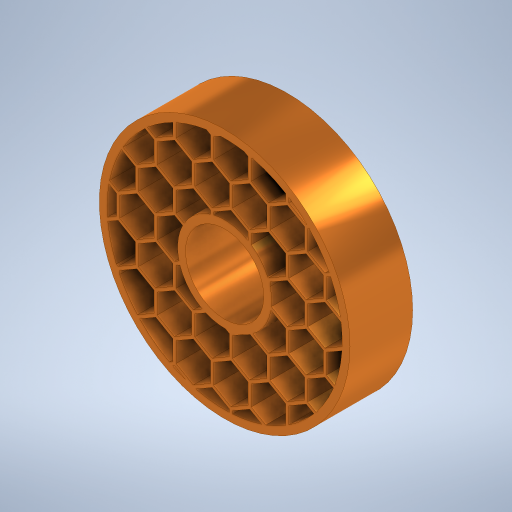
# Autodesk Inventor part: Idea3
Saved by Autodesk Inventor 2024.2 (Build 282272000, 272)
## iProperties
Created: 2025-07-14
Part Number: Idea3
Material: Generic
Document SubType Name: Modeling
Designer: Admin
Density: 1 g/cm^3
Appearance: Metal 1600F Hot
Author: Admin
Autodesk Inventor part; units mm, degrees
ref_plane "YZ Plane" through (0, 0, 0) normal (1, 0, 0) x (0, 1, 0)
ref_plane "XZ Plane" through (0, 0, 0) normal (0, 1, 0) x (-1, 0, 0)
ref_plane "XY Plane" through (0, 0, 0) normal (0, 0, 1) x (1, 0, 0)
sketch "Sketch1" plane through (0, 0, 0) normal (0, 0, 1) x (1, 0, 0)
  circle A0 centre (0, 0) radius 12.5
  circle A1 centre (0, 0) radius 40
  circle A2 centre (0, 0) radius 37.5
  circle A3 centre (0, 0) radius 15
  line L0 (0, 15) -> (0, 37.5) construction
  dimension "d2" = 75
  dimension "d3" = 30
  dimension "d0" = 25
  dimension "d1" = 80
  dimension "d4" = 22.5
  constraints: 4 coincident, 2 centre point, 2 end point, 2 vertical alignment, 1 vertical, 4 other
  measures "d0" diameter of A0
  measures "d1" diameter of A1
  measures "d4" distance of L0.start L0.end
extrude "Extrusion1" add sketch "Sketch1" along normal blind 20
sketch "Sketch2" plane through (0, 0, 20) normal (0, 0, 1) x (1, 0, 0)
  line L0 (40, -40) -> (-40, -40)
  line L1 (-40, -40) -> (-40, 40)
  line L2 (-40, 40) -> (40, 40)
  line L3 (40, 40) -> (40, -40)
  circle A0 centre (0, 0) radius 12.5 projected
  line L4 (40, -40) -> (-40, 40) construction
  line L5 (-40, -40) -> (40, 40) construction
  line L6 (-40, 40) -> (-64, 40) construction
  line L7 (-64, 40) -> (-64, -40) construction
  line L8 (-64, -40) -> (-40, -40)
  line L9 (-40, -40) -> (-40, 40)
  line L10 (-58, 40) -> (-52, 36.5359)
  line L11 (-52, 36.5359) -> (-52, 29.6077)
  line L12 (-58, 26.1436) -> (-64, 29.6077)
  line L13 (-64, 29.6077) -> (-64, 36.5359)
  line L14 (-64, 36.5359) -> (-58, 40)
  line L15 (-58, 33.0718) -> (-52, 22.6795) construction
  line L16 (-52, 29.6077) -> (-46, 26.1436)
  line L17 (-46, 26.1436) -> (-46, 19.2154)
  line L18 (-46, 19.2154) -> (-52, 15.7513)
  line L19 (-52, 15.7513) -> (-58, 19.2154)
  line L20 (-58, 19.2154) -> (-58, 26.1436)
  line L21 (-58, 26.1436) -> (-52, 29.6077)
  line L22 (-52.5, 36.2472) -> (-58, 39.4226)
  line L23 (-58, 39.4226) -> (-63.5, 36.2472)
  line L24 (-63.5, 36.2472) -> (-63.5, 29.8964)
  line L25 (-63.5, 29.8964) -> (-58, 26.7209)
  line L26 (-58, 26.7209) -> (-52.5, 29.8964)
  line L27 (-52.5, 29.8964) -> (-52.5, 36.2472)
  line L28 (-46.5, 25.8549) -> (-52, 29.0303)
  line L29 (-52, 29.0303) -> (-57.5, 25.8549)
  line L30 (-57.5, 25.8549) -> (-57.5, 19.5041)
  line L31 (-57.5, 19.5041) -> (-52, 16.3286)
  line L32 (-52, 16.3286) -> (-46.5, 19.5041)
  line L33 (-46.5, 19.5041) -> (-46.5, 25.8549)
  line L34 (-40.5, 36.2472) -> (-46, 39.4226)
  line L35 (-40.5, 29.8964) -> (-40.5, 36.2472)
  line L36 (-46, 39.4226) -> (-51.5, 36.2472)
  line L37 (-51.5, 36.2472) -> (-51.5, 29.8964)
  line L38 (-51.5, 29.8964) -> (-46, 26.7209)
  line L39 (-46, 26.7209) -> (-40.5, 29.8964)
  line L40 (-40, 29.0303) -> (-45.5, 25.8549)
  line L41 (-45.5, 25.8549) -> (-45.5, 19.5041)
  line L42 (-34.5, 25.8549) -> (-40, 29.0303)
  line L43 (-34.5, 19.5041) -> (-34.5, 25.8549)
  line L44 (-40, 16.3286) -> (-34.5, 19.5041)
  line L45 (-45.5, 19.5041) -> (-40, 16.3286)
  line L46 (-28.5, 36.2472) -> (-34, 39.4226)
  line L47 (-28.5, 29.8964) -> (-28.5, 36.2472)
  line L48 (-34, 39.4226) -> (-39.5, 36.2472)
  line L49 (-39.5, 36.2472) -> (-39.5, 29.8964)
  line L50 (-39.5, 29.8964) -> (-34, 26.7209)
  line L51 (-34, 26.7209) -> (-28.5, 29.8964)
  line L52 (-28, 29.0303) -> (-33.5, 25.8549)
  line L53 (-33.5, 25.8549) -> (-33.5, 19.5041)
  line L54 (-22.5, 25.8549) -> (-28, 29.0303)
  line L55 (-22.5, 19.5041) -> (-22.5, 25.8549)
  line L56 (-28, 16.3286) -> (-22.5, 19.5041)
  line L57 (-33.5, 19.5041) -> (-28, 16.3286)
  line L58 (-16.5, 36.2472) -> (-22, 39.4226)
  line L59 (-16.5, 29.8964) -> (-16.5, 36.2472)
  line L60 (-22, 39.4226) -> (-27.5, 36.2472)
  line L61 (-27.5, 36.2472) -> (-27.5, 29.8964)
  line L62 (-27.5, 29.8964) -> (-22, 26.7209)
  line L63 (-22, 26.7209) -> (-16.5, 29.8964)
  line L64 (-16, 29.0303) -> (-21.5, 25.8549)
  line L65 (-21.5, 25.8549) -> (-21.5, 19.5041)
  line L66 (-10.5, 25.8549) -> (-16, 29.0303)
  line L67 (-10.5, 19.5041) -> (-10.5, 25.8549)
  line L68 (-16, 16.3286) -> (-10.5, 19.5041)
  line L69 (-21.5, 19.5041) -> (-16, 16.3286)
  line L70 (-4.5, 36.2472) -> (-10, 39.4226)
  line L71 (-4.5, 29.8964) -> (-4.5, 36.2472)
  line L72 (-10, 39.4226) -> (-15.5, 36.2472)
  line L73 (-15.5, 36.2472) -> (-15.5, 29.8964)
  line L74 (-15.5, 29.8964) -> (-10, 26.7209)
  line L75 (-10, 26.7209) -> (-4.5, 29.8964)
  line L76 (-4, 29.0303) -> (-9.5, 25.8549)
  line L77 (-9.5, 25.8549) -> (-9.5, 19.5041)
  line L78 (1.5, 25.8549) -> (-4, 29.0303)
  line L79 (1.5, 19.5041) -> (1.5, 25.8549)
  line L80 (-4, 16.3286) -> (1.5, 19.5041)
  line L81 (-9.5, 19.5041) -> (-4, 16.3286)
  line L82 (7.5, 36.2472) -> (2, 39.4226)
  line L83 (7.5, 29.8964) -> (7.5, 36.2472)
  line L84 (2, 39.4226) -> (-3.5, 36.2472)
  line L85 (-3.5, 36.2472) -> (-3.5, 29.8964)
  line L86 (-3.5, 29.8964) -> (2, 26.7209)
  line L87 (2, 26.7209) -> (7.5, 29.8964)
  line L88 (8, 29.0303) -> (2.5, 25.8549)
  line L89 (2.5, 25.8549) -> (2.5, 19.5041)
  line L90 (13.5, 25.8549) -> (8, 29.0303)
  line L91 (13.5, 19.5041) -> (13.5, 25.8549)
  line L92 (8, 16.3286) -> (13.5, 19.5041)
  line L93 (2.5, 19.5041) -> (8, 16.3286)
  line L94 (19.5, 36.2472) -> (14, 39.4226)
  line L95 (19.5, 29.8964) -> (19.5, 36.2472)
  line L96 (14, 39.4226) -> (8.5, 36.2472)
  line L97 (8.5, 36.2472) -> (8.5, 29.8964)
  line L98 (8.5, 29.8964) -> (14, 26.7209)
  line L99 (14, 26.7209) -> (19.5, 29.8964)
  line L100 (20, 29.0303) -> (14.5, 25.8549)
  line L101 (14.5, 25.8549) -> (14.5, 19.5041)
  line L102 (25.5, 25.8549) -> (20, 29.0303)
  line L103 (25.5, 19.5041) -> (25.5, 25.8549)
  line L104 (20, 16.3286) -> (25.5, 19.5041)
  line L105 (14.5, 19.5041) -> (20, 16.3286)
  line L106 (31.5, 36.2472) -> (26, 39.4226)
  line L107 (31.5, 29.8964) -> (31.5, 36.2472)
  line L108 (26, 39.4226) -> (20.5, 36.2472)
  line L109 (20.5, 36.2472) -> (20.5, 29.8964)
  line L110 (20.5, 29.8964) -> (26, 26.7209)
  line L111 (26, 26.7209) -> (31.5, 29.8964)
  line L112 (32, 29.0303) -> (26.5, 25.8549)
  line L113 (26.5, 25.8549) -> (26.5, 19.5041)
  line L114 (37.5, 25.8549) -> (32, 29.0303)
  line L115 (37.5, 19.5041) -> (37.5, 25.8549)
  line L116 (32, 16.3286) -> (37.5, 19.5041)
  line L117 (26.5, 19.5041) -> (32, 16.3286)
  line L118 (43.5, 36.2472) -> (38, 39.4226)
  line L119 (43.5, 29.8964) -> (43.5, 36.2472)
  line L120 (38, 39.4226) -> (32.5, 36.2472)
  line L121 (32.5, 36.2472) -> (32.5, 29.8964)
  line L122 (32.5, 29.8964) -> (38, 26.7209)
  line L123 (38, 26.7209) -> (43.5, 29.8964)
  line L124 (44, 29.0303) -> (38.5, 25.8549)
  line L125 (38.5, 25.8549) -> (38.5, 19.5041)
  line L126 (49.5, 25.8549) -> (44, 29.0303)
  line L127 (49.5, 19.5041) -> (49.5, 25.8549)
  line L128 (44, 16.3286) -> (49.5, 19.5041)
  line L129 (38.5, 19.5041) -> (44, 16.3286)
  line L130 (-52.5, 15.4626) -> (-58, 18.638)
  line L131 (-52.5, 9.1118) -> (-52.5, 15.4626)
  line L132 (-58, 18.638) -> (-63.5, 15.4626)
  line L133 (-63.5, 15.4626) -> (-63.5, 9.1118)
  line L134 (-63.5, 9.1118) -> (-58, 5.9363)
  line L135 (-58, 5.9363) -> (-52.5, 9.1118)
  line L136 (-52, 8.2457) -> (-57.5, 5.0703)
  line L137 (-57.5, 5.0703) -> (-57.5, -1.2805)
  line L138 (-46.5, 5.0703) -> (-52, 8.2457)
  line L139 (-46.5, -1.2805) -> (-46.5, 5.0703)
  line L140 (-52, -4.456) -> (-46.5, -1.2805)
  line L141 (-57.5, -1.2805) -> (-52, -4.456)
  line L142 (-40.5, 15.4626) -> (-46, 18.638)
  line L143 (-40.5, 9.1118) -> (-40.5, 15.4626)
  line L144 (-46, 18.638) -> (-51.5, 15.4626)
  line L145 (-51.5, 15.4626) -> (-51.5, 9.1118)
  line L146 (-51.5, 9.1118) -> (-46, 5.9363)
  line L147 (-46, 5.9363) -> (-40.5, 9.1118)
  line L148 (-40, 8.2457) -> (-45.5, 5.0703)
  line L149 (-45.5, 5.0703) -> (-45.5, -1.2805)
  line L150 (-34.5, 5.0703) -> (-40, 8.2457)
  line L151 (-34.5, -1.2805) -> (-34.5, 5.0703)
  line L152 (-40, -4.456) -> (-34.5, -1.2805)
  line L153 (-45.5, -1.2805) -> (-40, -4.456)
  line L154 (-28.5, 15.4626) -> (-34, 18.638)
  line L155 (-28.5, 9.1118) -> (-28.5, 15.4626)
  line L156 (-34, 18.638) -> (-39.5, 15.4626)
  line L157 (-39.5, 15.4626) -> (-39.5, 9.1118)
  line L158 (-39.5, 9.1118) -> (-34, 5.9363)
  line L159 (-34, 5.9363) -> (-28.5, 9.1118)
  line L160 (-28, 8.2457) -> (-33.5, 5.0703)
  line L161 (-33.5, 5.0703) -> (-33.5, -1.2805)
  line L162 (-22.5, 5.0703) -> (-28, 8.2457)
  line L163 (-22.5, -1.2805) -> (-22.5, 5.0703)
  line L164 (-28, -4.456) -> (-22.5, -1.2805)
  line L165 (-33.5, -1.2805) -> (-28, -4.456)
  line L166 (-16.5, 15.4626) -> (-22, 18.638)
  line L167 (-16.5, 9.1118) -> (-16.5, 15.4626)
  line L168 (-22, 18.638) -> (-27.5, 15.4626)
  line L169 (-27.5, 15.4626) -> (-27.5, 9.1118)
  line L170 (-27.5, 9.1118) -> (-22, 5.9363)
  line L171 (-22, 5.9363) -> (-16.5, 9.1118)
  line L172 (-16, 8.2457) -> (-21.5, 5.0703)
  line L173 (-21.5, 5.0703) -> (-21.5, -1.2805)
  line L174 (-10.5, 5.0703) -> (-16, 8.2457)
  line L175 (-10.5, -1.2805) -> (-10.5, 5.0703)
  line L176 (-16, -4.456) -> (-10.5, -1.2805)
  line L177 (-21.5, -1.2805) -> (-16, -4.456)
  line L178 (-4.5, 15.4626) -> (-10, 18.638)
  line L179 (-4.5, 9.1118) -> (-4.5, 15.4626)
  line L180 (-10, 18.638) -> (-15.5, 15.4626)
  line L181 (-15.5, 15.4626) -> (-15.5, 9.1118)
  line L182 (-15.5, 9.1118) -> (-10, 5.9363)
  line L183 (-10, 5.9363) -> (-4.5, 9.1118)
  line L184 (-4, 8.2457) -> (-9.5, 5.0703)
  line L185 (-9.5, 5.0703) -> (-9.5, -1.2805)
  line L186 (1.5, 5.0703) -> (-4, 8.2457)
  line L187 (1.5, -1.2805) -> (1.5, 5.0703)
  line L188 (-4, -4.456) -> (1.5, -1.2805)
  line L189 (-9.5, -1.2805) -> (-4, -4.456)
  line L190 (7.5, 15.4626) -> (2, 18.638)
  line L191 (7.5, 9.1118) -> (7.5, 15.4626)
  line L192 (2, 18.638) -> (-3.5, 15.4626)
  line L193 (-3.5, 15.4626) -> (-3.5, 9.1118)
  line L194 (-3.5, 9.1118) -> (2, 5.9363)
  line L195 (2, 5.9363) -> (7.5, 9.1118)
  line L196 (8, 8.2457) -> (2.5, 5.0703)
  line L197 (2.5, 5.0703) -> (2.5, -1.2805)
  line L198 (13.5, 5.0703) -> (8, 8.2457)
  line L199 (13.5, -1.2805) -> (13.5, 5.0703)
  line L200 (8, -4.456) -> (13.5, -1.2805)
  line L201 (2.5, -1.2805) -> (8, -4.456)
  line L202 (19.5, 15.4626) -> (14, 18.638)
  line L203 (19.5, 9.1118) -> (19.5, 15.4626)
  line L204 (14, 18.638) -> (8.5, 15.4626)
  line L205 (8.5, 15.4626) -> (8.5, 9.1118)
  line L206 (8.5, 9.1118) -> (14, 5.9363)
  line L207 (14, 5.9363) -> (19.5, 9.1118)
  line L208 (20, 8.2457) -> (14.5, 5.0703)
  line L209 (14.5, 5.0703) -> (14.5, -1.2805)
  line L210 (25.5, 5.0703) -> (20, 8.2457)
  line L211 (25.5, -1.2805) -> (25.5, 5.0703)
  line L212 (20, -4.456) -> (25.5, -1.2805)
  line L213 (14.5, -1.2805) -> (20, -4.456)
  line L214 (31.5, 15.4626) -> (26, 18.638)
  line L215 (31.5, 9.1118) -> (31.5, 15.4626)
  line L216 (26, 18.638) -> (20.5, 15.4626)
  line L217 (20.5, 15.4626) -> (20.5, 9.1118)
  line L218 (20.5, 9.1118) -> (26, 5.9363)
  line L219 (26, 5.9363) -> (31.5, 9.1118)
  line L220 (32, 8.2457) -> (26.5, 5.0703)
  line L221 (26.5, 5.0703) -> (26.5, -1.2805)
  line L222 (37.5, 5.0703) -> (32, 8.2457)
  line L223 (37.5, -1.2805) -> (37.5, 5.0703)
  line L224 (32, -4.456) -> (37.5, -1.2805)
  line L225 (26.5, -1.2805) -> (32, -4.456)
  line L226 (43.5, 15.4626) -> (38, 18.638)
  line L227 (43.5, 9.1118) -> (43.5, 15.4626)
  line L228 (38, 18.638) -> (32.5, 15.4626)
  line L229 (32.5, 15.4626) -> (32.5, 9.1118)
  line L230 (32.5, 9.1118) -> (38, 5.9363)
  line L231 (38, 5.9363) -> (43.5, 9.1118)
  line L232 (44, 8.2457) -> (38.5, 5.0703)
  line L233 (38.5, 5.0703) -> (38.5, -1.2805)
  line L234 (49.5, 5.0703) -> (44, 8.2457)
  line L235 (49.5, -1.2805) -> (49.5, 5.0703)
  line L236 (44, -4.456) -> (49.5, -1.2805)
  line L237 (38.5, -1.2805) -> (44, -4.456)
  line L238 (-52.5, -5.322) -> (-58, -2.1466)
  line L239 (-52.5, -11.6728) -> (-52.5, -5.322)
  line L240 (-58, -2.1466) -> (-63.5, -5.322)
  line L241 (-63.5, -5.322) -> (-63.5, -11.6728)
  line L242 (-63.5, -11.6728) -> (-58, -14.8483)
  line L243 (-58, -14.8483) -> (-52.5, -11.6728)
  line L244 (-52, -12.5389) -> (-57.5, -15.7143)
  line L245 (-57.5, -15.7143) -> (-57.5, -22.0652)
  line L246 (-46.5, -15.7143) -> (-52, -12.5389)
  line L247 (-46.5, -22.0652) -> (-46.5, -15.7143)
  line L248 (-52, -25.2406) -> (-46.5, -22.0652)
  line L249 (-57.5, -22.0652) -> (-52, -25.2406)
  line L250 (-40.5, -5.322) -> (-46, -2.1466)
  line L251 (-40.5, -11.6728) -> (-40.5, -5.322)
  line L252 (-46, -2.1466) -> (-51.5, -5.322)
  line L253 (-51.5, -5.322) -> (-51.5, -11.6728)
  line L254 (-51.5, -11.6728) -> (-46, -14.8483)
  line L255 (-46, -14.8483) -> (-40.5, -11.6728)
  line L256 (-40, -12.5389) -> (-45.5, -15.7143)
  line L257 (-45.5, -15.7143) -> (-45.5, -22.0652)
  line L258 (-34.5, -15.7143) -> (-40, -12.5389)
  line L259 (-34.5, -22.0652) -> (-34.5, -15.7143)
  line L260 (-40, -25.2406) -> (-34.5, -22.0652)
  line L261 (-45.5, -22.0652) -> (-40, -25.2406)
  line L262 (-28.5, -5.322) -> (-34, -2.1466)
  line L263 (-28.5, -11.6728) -> (-28.5, -5.322)
  line L264 (-34, -2.1466) -> (-39.5, -5.322)
  line L265 (-39.5, -5.322) -> (-39.5, -11.6728)
  line L266 (-39.5, -11.6728) -> (-34, -14.8483)
  line L267 (-34, -14.8483) -> (-28.5, -11.6728)
  line L268 (-28, -12.5389) -> (-33.5, -15.7143)
  line L269 (-33.5, -15.7143) -> (-33.5, -22.0652)
  line L270 (-22.5, -15.7143) -> (-28, -12.5389)
  line L271 (-22.5, -22.0652) -> (-22.5, -15.7143)
  line L272 (-28, -25.2406) -> (-22.5, -22.0652)
  line L273 (-33.5, -22.0652) -> (-28, -25.2406)
  line L274 (-16.5, -5.322) -> (-22, -2.1466)
  line L275 (-16.5, -11.6728) -> (-16.5, -5.322)
  line L276 (-22, -2.1466) -> (-27.5, -5.322)
  line L277 (-27.5, -5.322) -> (-27.5, -11.6728)
  line L278 (-27.5, -11.6728) -> (-22, -14.8483)
  line L279 (-22, -14.8483) -> (-16.5, -11.6728)
  line L280 (-16, -12.5389) -> (-21.5, -15.7143)
  line L281 (-21.5, -15.7143) -> (-21.5, -22.0652)
  line L282 (-10.5, -15.7143) -> (-16, -12.5389)
  line L283 (-10.5, -22.0652) -> (-10.5, -15.7143)
  line L284 (-16, -25.2406) -> (-10.5, -22.0652)
  line L285 (-21.5, -22.0652) -> (-16, -25.2406)
  line L286 (-4.5, -5.322) -> (-10, -2.1466)
  line L287 (-4.5, -11.6728) -> (-4.5, -5.322)
  line L288 (-10, -2.1466) -> (-15.5, -5.322)
  line L289 (-15.5, -5.322) -> (-15.5, -11.6728)
  line L290 (-15.5, -11.6728) -> (-10, -14.8483)
  line L291 (-10, -14.8483) -> (-4.5, -11.6728)
  line L292 (-4, -12.5389) -> (-9.5, -15.7143)
  line L293 (-9.5, -15.7143) -> (-9.5, -22.0652)
  line L294 (1.5, -15.7143) -> (-4, -12.5389)
  line L295 (1.5, -22.0652) -> (1.5, -15.7143)
  line L296 (-4, -25.2406) -> (1.5, -22.0652)
  line L297 (-9.5, -22.0652) -> (-4, -25.2406)
  line L298 (7.5, -5.322) -> (2, -2.1466)
  line L299 (7.5, -11.6728) -> (7.5, -5.322)
  line L300 (2, -2.1466) -> (-3.5, -5.322)
  line L301 (-3.5, -5.322) -> (-3.5, -11.6728)
  line L302 (-3.5, -11.6728) -> (2, -14.8483)
  line L303 (2, -14.8483) -> (7.5, -11.6728)
  line L304 (8, -12.5389) -> (2.5, -15.7143)
  line L305 (2.5, -15.7143) -> (2.5, -22.0652)
  line L306 (13.5, -15.7143) -> (8, -12.5389)
  line L307 (13.5, -22.0652) -> (13.5, -15.7143)
  line L308 (8, -25.2406) -> (13.5, -22.0652)
  line L309 (2.5, -22.0652) -> (8, -25.2406)
  line L310 (19.5, -5.322) -> (14, -2.1466)
  line L311 (19.5, -11.6728) -> (19.5, -5.322)
  line L312 (14, -2.1466) -> (8.5, -5.322)
  line L313 (8.5, -5.322) -> (8.5, -11.6728)
  line L314 (8.5, -11.6728) -> (14, -14.8483)
  line L315 (14, -14.8483) -> (19.5, -11.6728)
  line L316 (20, -12.5389) -> (14.5, -15.7143)
  line L317 (14.5, -15.7143) -> (14.5, -22.0652)
  line L318 (25.5, -15.7143) -> (20, -12.5389)
  line L319 (25.5, -22.0652) -> (25.5, -15.7143)
  line L320 (20, -25.2406) -> (25.5, -22.0652)
  line L321 (14.5, -22.0652) -> (20, -25.2406)
  line L322 (31.5, -5.322) -> (26, -2.1466)
  line L323 (31.5, -11.6728) -> (31.5, -5.322)
  line L324 (26, -2.1466) -> (20.5, -5.322)
  line L325 (20.5, -5.322) -> (20.5, -11.6728)
  line L326 (20.5, -11.6728) -> (26, -14.8483)
  line L327 (26, -14.8483) -> (31.5, -11.6728)
  line L328 (32, -12.5389) -> (26.5, -15.7143)
  line L329 (26.5, -15.7143) -> (26.5, -22.0652)
  line L330 (37.5, -15.7143) -> (32, -12.5389)
  line L331 (37.5, -22.0652) -> (37.5, -15.7143)
  line L332 (32, -25.2406) -> (37.5, -22.0652)
  line L333 (26.5, -22.0652) -> (32, -25.2406)
  line L334 (43.5, -5.322) -> (38, -2.1466)
  line L335 (43.5, -11.6728) -> (43.5, -5.322)
  line L336 (38, -2.1466) -> (32.5, -5.322)
  line L337 (32.5, -5.322) -> (32.5, -11.6728)
  line L338 (32.5, -11.6728) -> (38, -14.8483)
  line L339 (38, -14.8483) -> (43.5, -11.6728)
  line L340 (44, -12.5389) -> (38.5, -15.7143)
  line L341 (38.5, -15.7143) -> (38.5, -22.0652)
  line L342 (49.5, -15.7143) -> (44, -12.5389)
  line L343 (49.5, -22.0652) -> (49.5, -15.7143)
  line L344 (44, -25.2406) -> (49.5, -22.0652)
  line L345 (38.5, -22.0652) -> (44, -25.2406)
  line L346 (-52.5, -26.1066) -> (-58, -22.9312)
  line L347 (-52.5, -32.4575) -> (-52.5, -26.1066)
  line L348 (-58, -22.9312) -> (-63.5, -26.1066)
  line L349 (-63.5, -26.1066) -> (-63.5, -32.4575)
  line L350 (-63.5, -32.4575) -> (-58, -35.6329)
  line L351 (-58, -35.6329) -> (-52.5, -32.4575)
  line L352 (-52, -33.3235) -> (-57.5, -36.4989)
  line L353 (-57.5, -36.4989) -> (-57.5, -42.8498)
  line L354 (-46.5, -36.4989) -> (-52, -33.3235)
  line L355 (-46.5, -42.8498) -> (-46.5, -36.4989)
  line L356 (-52, -46.0252) -> (-46.5, -42.8498)
  line L357 (-57.5, -42.8498) -> (-52, -46.0252)
  line L358 (-40.5, -26.1066) -> (-46, -22.9312)
  line L359 (-40.5, -32.4575) -> (-40.5, -26.1066)
  line L360 (-46, -22.9312) -> (-51.5, -26.1066)
  line L361 (-51.5, -26.1066) -> (-51.5, -32.4575)
  line L362 (-51.5, -32.4575) -> (-46, -35.6329)
  line L363 (-46, -35.6329) -> (-40.5, -32.4575)
  line L364 (-40, -33.3235) -> (-45.5, -36.4989)
  line L365 (-45.5, -36.4989) -> (-45.5, -42.8498)
  line L366 (-34.5, -36.4989) -> (-40, -33.3235)
  line L367 (-34.5, -42.8498) -> (-34.5, -36.4989)
  line L368 (-40, -46.0252) -> (-34.5, -42.8498)
  line L369 (-45.5, -42.8498) -> (-40, -46.0252)
  line L370 (-28.5, -26.1066) -> (-34, -22.9312)
  line L371 (-28.5, -32.4575) -> (-28.5, -26.1066)
  line L372 (-34, -22.9312) -> (-39.5, -26.1066)
  line L373 (-39.5, -26.1066) -> (-39.5, -32.4575)
  line L374 (-39.5, -32.4575) -> (-34, -35.6329)
  line L375 (-34, -35.6329) -> (-28.5, -32.4575)
  line L376 (-28, -33.3235) -> (-33.5, -36.4989)
  line L377 (-33.5, -36.4989) -> (-33.5, -42.8498)
  line L378 (-22.5, -36.4989) -> (-28, -33.3235)
  line L379 (-22.5, -42.8498) -> (-22.5, -36.4989)
  line L380 (-28, -46.0252) -> (-22.5, -42.8498)
  line L381 (-33.5, -42.8498) -> (-28, -46.0252)
  line L382 (-16.5, -26.1066) -> (-22, -22.9312)
  line L383 (-16.5, -32.4575) -> (-16.5, -26.1066)
  line L384 (-22, -22.9312) -> (-27.5, -26.1066)
  line L385 (-27.5, -26.1066) -> (-27.5, -32.4575)
  line L386 (-27.5, -32.4575) -> (-22, -35.6329)
  line L387 (-22, -35.6329) -> (-16.5, -32.4575)
  line L388 (-16, -33.3235) -> (-21.5, -36.4989)
  line L389 (-21.5, -36.4989) -> (-21.5, -42.8498)
  line L390 (-10.5, -36.4989) -> (-16, -33.3235)
  line L391 (-10.5, -42.8498) -> (-10.5, -36.4989)
  line L392 (-16, -46.0252) -> (-10.5, -42.8498)
  line L393 (-21.5, -42.8498) -> (-16, -46.0252)
  line L394 (-4.5, -26.1066) -> (-10, -22.9312)
  line L395 (-4.5, -32.4575) -> (-4.5, -26.1066)
  line L396 (-10, -22.9312) -> (-15.5, -26.1066)
  line L397 (-15.5, -26.1066) -> (-15.5, -32.4575)
  line L398 (-15.5, -32.4575) -> (-10, -35.6329)
  line L399 (-10, -35.6329) -> (-4.5, -32.4575)
  line L400 (-4, -33.3235) -> (-9.5, -36.4989)
  line L401 (-9.5, -36.4989) -> (-9.5, -42.8498)
  line L402 (1.5, -36.4989) -> (-4, -33.3235)
  line L403 (1.5, -42.8498) -> (1.5, -36.4989)
  line L404 (-4, -46.0252) -> (1.5, -42.8498)
  line L405 (-9.5, -42.8498) -> (-4, -46.0252)
  line L406 (7.5, -26.1066) -> (2, -22.9312)
  line L407 (7.5, -32.4575) -> (7.5, -26.1066)
  line L408 (2, -22.9312) -> (-3.5, -26.1066)
  line L409 (-3.5, -26.1066) -> (-3.5, -32.4575)
  line L410 (-3.5, -32.4575) -> (2, -35.6329)
  line L411 (2, -35.6329) -> (7.5, -32.4575)
  line L412 (8, -33.3235) -> (2.5, -36.4989)
  line L413 (2.5, -36.4989) -> (2.5, -42.8498)
  line L414 (13.5, -36.4989) -> (8, -33.3235)
  line L415 (13.5, -42.8498) -> (13.5, -36.4989)
  line L416 (8, -46.0252) -> (13.5, -42.8498)
  line L417 (2.5, -42.8498) -> (8, -46.0252)
  line L418 (19.5, -26.1066) -> (14, -22.9312)
  line L419 (19.5, -32.4575) -> (19.5, -26.1066)
  line L420 (14, -22.9312) -> (8.5, -26.1066)
  line L421 (8.5, -26.1066) -> (8.5, -32.4575)
  line L422 (8.5, -32.4575) -> (14, -35.6329)
  line L423 (14, -35.6329) -> (19.5, -32.4575)
  line L424 (20, -33.3235) -> (14.5, -36.4989)
  line L425 (14.5, -36.4989) -> (14.5, -42.8498)
  line L426 (25.5, -36.4989) -> (20, -33.3235)
  line L427 (25.5, -42.8498) -> (25.5, -36.4989)
  line L428 (20, -46.0252) -> (25.5, -42.8498)
  line L429 (14.5, -42.8498) -> (20, -46.0252)
  line L430 (31.5, -26.1066) -> (26, -22.9312)
  line L431 (31.5, -32.4575) -> (31.5, -26.1066)
  line L432 (26, -22.9312) -> (20.5, -26.1066)
  line L433 (20.5, -26.1066) -> (20.5, -32.4575)
  line L434 (20.5, -32.4575) -> (26, -35.6329)
  line L435 (26, -35.6329) -> (31.5, -32.4575)
  line L436 (32, -33.3235) -> (26.5, -36.4989)
  line L437 (26.5, -36.4989) -> (26.5, -42.8498)
  line L438 (37.5, -36.4989) -> (32, -33.3235)
  line L439 (37.5, -42.8498) -> (37.5, -36.4989)
  line L440 (32, -46.0252) -> (37.5, -42.8498)
  line L441 (26.5, -42.8498) -> (32, -46.0252)
  line L442 (43.5, -26.1066) -> (38, -22.9312)
  line L443 (43.5, -32.4575) -> (43.5, -26.1066)
  line L444 (38, -22.9312) -> (32.5, -26.1066)
  line L445 (32.5, -26.1066) -> (32.5, -32.4575)
  line L446 (32.5, -32.4575) -> (38, -35.6329)
  line L447 (38, -35.6329) -> (43.5, -32.4575)
  line L448 (44, -33.3235) -> (38.5, -36.4989)
  line L449 (38.5, -36.4989) -> (38.5, -42.8498)
  line L450 (49.5, -36.4989) -> (44, -33.3235)
  line L451 (49.5, -42.8498) -> (49.5, -36.4989)
  line L452 (44, -46.0252) -> (49.5, -42.8498)
  line L453 (38.5, -42.8498) -> (44, -46.0252)
  circle A1 centre (0, 0) radius 37.5
  point P0 (-32.4052, 18.872)
  point P1 (-32.8969, 18.0012)
  point P2 (-36.7388, 7.5176)
  point P3 (-36.9364, 6.477)
  point P4 (-37.3841, -2.9457)
  point P5 (-37.2816, -4.0412)
  point P6 (-34.5768, -14.5152)
  point P7 (-33.5, -16.8523)
  point P8 (-27.8253, -25.1397)
  point P9 (-27.1272, -25.8914)
  point P10 (-17.6187, -33.1033)
  point P11 (-16.5587, -33.6461)
  point P12 (-12.4504, -35.3728)
  point P13 (-9.234, -36.3453)
  point P14 (1.5, -37.47)
  point P15 (2.5, -37.4166)
  point P16 (11.8853, -35.5667)
  point P17 (13.1254, -35.128)
  point P18 (19.5, -32.0312)
  point P19 (20.5, -31.4006)
  point P20 (28.4986, -24.3737)
  point P21 (29.1476, -23.5938)
  point P22 (34.7398, -14.1207)
  point P23 (35.108, -13.1786)
  point P24 (37.4177, -2.4827)
  point P25 (37.4777, -1.2934)
  point P26 (37.1255, 5.2865)
  point P27 (36.922, 6.5587)
  point P28 (33.8109, 16.2195)
  point P29 (33.3655, 17.117)
  point P30 (26.9258, 26.1008)
  point P31 (26.1954, 26.8338)
  point P32 (20.5, 31.4006)
  point P33 (19.5, 32.0312)
  point P34 (8.8396, 36.4433)
  point P35 (6.2339, 36.9782)
  point P36 (-1.3737, 37.4748)
  point P37 (-5.8694, 37.0378)
  point P38 (-15.5, 34.1467)
  point P39 (-16.5, 33.6749)
  point P40 (-24.6563, 28.2545)
  point P41 (-25.4391, 27.5518)
  point P42 (-11.2292, 5.4913)
  point P43 (-10.7541, 6.3717)
  point P44 (-4.5, 11.6619)
  point P45 (-3.5, 12)
  point P46 (7.5, 10)
  point P47 (8.5, 9.1652)
  point P48 (8.6462, 9.0273)
  point P49 (10.4793, 6.8143)
  point P50 (12.3476, -1.9459)
  point P51 (12.0667, -3.2628)
  point P52 (8.5, -9.1652)
  point P53 (7.5, -10)
  point P54 (-2.5074, -12.2459)
  point P55 (-4.5, -11.6619)
  point P56 (-12.0485, -3.3293)
  point P57 (-12.2845, -2.3108)
  dimension "d7" = 80
  dimension "d8" = 24
  dimension "d15" = 6
  dimension "d16" = 6.9282
  dimension "d17" = 12
  dimension "d18" = 0.5
  dimension "d19" = 0.5
  dimension "d22" = 12
  dimension "d25" = 20.7846
  constraints: 908 end point, 4 parallel, 3 horizontal, 2 coincident, 2 midpoint, 2 perpendicular, 1 point on line, 1 vertical, 874 other
  measures "d7" distance of L1.end L2.end
  measures "d8" distance of L8.end L7.end
  measures "d15" distance from line of L7 L15.start
  measures "d16" distance from line of L6 L15.start
  measures "d17" distance of L15.start L15.end
  measures "d18" distance between parallel lines of L10 L22
  measures "d19" distance between parallel lines of L16 L28
  measures "d22" distance of L22.start L34.start
  measures "d25" distance of L22.start L130.start
extrude "Extrusion2" add sketch "Sketch2" against normal blind 20 contours A1 L403 L402 L400 L390 L388 L387 L383 L382 L384 L272 L271 L270 L268 L269 L266 L267 L263 L262 L264 L152 L151 L150 L158 L159 L155 L154 L57 L56 L55 L54 L62 L63 L59 L73 L74 L75 L71 L70 L84 L85 L86 L87 L83 L82 L96 L97 L98 L99 L95 L109 L110 L111 L112 L113 L117 L116 L228 L229 L230 L222 L220 L221 L225 L224 L336 L337 L338 L330 L328 L329 L333 L430 L432 L433 L419 L418 L420 L421 L422 L414 L412 L413
body "Solid1"
